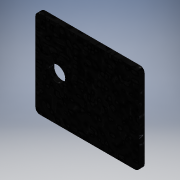
# Autodesk Inventor part: Neje_Base_slide_x
Saved by Autodesk Inventor 2019.4 (Build 234330000, 330)
## iProperties
Created: 2021-04-08
Part Number: Neje_Base_slide_x
Material: Generic
Document SubType Name: Modeling
Designer: diederichbenedict
Density: 1 g/cm^3
Appearance: Black
Author: diederichbenedict
Autodesk Inventor part; units mm, degrees
ref_plane "YZ Plane" through (0, 0, 0) normal (1, 0, 0) x (0, 1, 0)
ref_plane "XZ Plane" through (0, 0, 0) normal (0, 1, 0) x (-1, 0, 0)
ref_plane "XY Plane" through (0, 0, 0) normal (0, 0, 1) x (1, 0, 0)
sketch "Sketch1" plane through (0, 0, 0) normal (0, 0, 1) x (1, 0, 0)
  line L0 (21.0847, 68.8136) -> (-66.9153, 68.8136)
  line L1 (-70.9153, 72.8136) -> (-70.9153, 145.8136)
  line L2 (-66.9153, 149.8136) -> (21.0847, 149.8136)
  line L3 (25.0847, 145.8136) -> (25.0847, 72.8136)
  line L4 (4.925, 0) -> (4.925, 205.34) projected
  line L5 (-25.075, 0) -> (-25.075, 205.34) projected
  arc A0 (-66.9153, 149.8136) -> (-70.9153, 145.8136) centre (-66.9153, 145.8136) ccw
  arc A1 (25.0847, 145.8136) -> (21.0847, 149.8136) centre (21.0847, 145.8136) ccw
  arc A2 (21.0847, 68.8136) -> (25.0847, 72.8136) centre (21.0847, 72.8136) ccw
  arc A3 (-70.9153, 72.8136) -> (-66.9153, 68.8136) centre (-66.9153, 72.8136) ccw
  point P0 (0, 0)
  dimension "d0" = 96
  dimension "d1" = 81
  dimension "d2" = 4
  constraints: 8 end point, 8 point on circle, 8 tangent, 4 centre point, 3 equal radius, 2 parallel, 1 horizontal, 1 perpendicular
  measures "d0" distance between parallel lines of L3 L1
  measures "d1" distance between parallel lines of L2 L0
  measures "d2" radius of A0
extrude "Extrusion1" add sketch "Sketch1" along normal blind 4.7
sketch "Sketch2" plane through (0, 0, 4.7) normal (0, 0, 1) x (1, 0, 0)
  line L0 (21.0847, 149.8136) -> (-66.9153, 149.8136) projected
  arc A0 (-66.9153, 149.8136) -> (-70.9153, 145.8136) centre (-66.9153, 145.8136) ccw projected
  line L1 (-70.9153, 145.8136) -> (-70.9153, 72.8136) projected
  arc A1 (-70.9153, 72.8136) -> (-66.9153, 68.8136) centre (-66.9153, 72.8136) ccw projected
  line L2 (-66.9153, 68.8136) -> (21.0847, 68.8136) projected
  arc A2 (21.0847, 68.8136) -> (25.0847, 72.8136) centre (21.0847, 72.8136) ccw projected
  line L3 (25.0847, 72.8136) -> (25.0847, 145.8136) projected
  arc A3 (25.0847, 145.8136) -> (21.0847, 149.8136) centre (21.0847, 145.8136) ccw projected
  circle A4 centre (-50.9153, 109.3136) radius 7.448
  point P0 (0, 0)
  dimension "d5" = 20
  constraints: 1 centre point
  measures "d5" distance from line of A4.centre L1
extrude "Extrusion2" cut sketch "Sketch2" against normal through all contours A4
body "Solid1"
